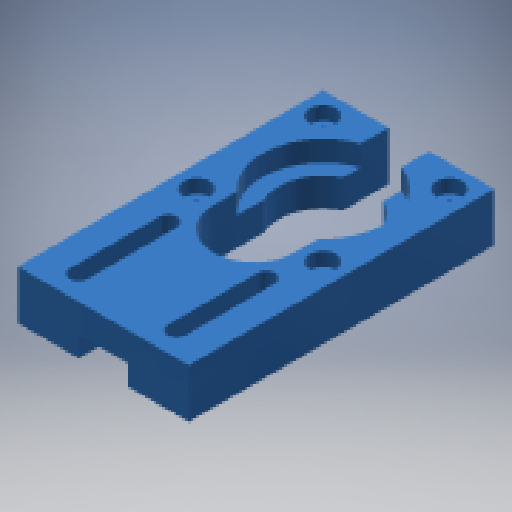
# Autodesk Inventor part: 24_0497_008
Saved by Autodesk Inventor 2024.3 (Build 283343000, 343)
## iProperties
Created: 2024-06-11
Part Number: 24_0497_008
Material: Allgemein
Document SubType Name: Modeling
Designer: Vogel
Density: 1 g/cm^3
Appearance: Cyan
Author: Vogel
Autodesk Inventor part; units mm, degrees
ref_plane "YZ Plane" through (0, 0, 0) normal (1, 0, 0) x (0, 1, 0)
ref_plane "XZ Plane" through (0, 0, 0) normal (0, 1, 0) x (-1, 0, 0)
ref_plane "XY Plane" through (0, 0, 0) normal (0, 0, 1) x (1, 0, 0)
sketch "Skizze1" plane through (0, 0, 0) normal (0, 0, 1) x (1, 0, 0)
  line L0 (-29.4, 0) -> (29.4, 0) projected
  line L1 (0, -69) -> (0, 36) projected
  line L2 (21, -54) -> (-21, -54)
  line L3 (-21, -54) -> (-21, 21)
  line L4 (-21, 21) -> (21, 21)
  line L5 (21, 21) -> (21, -54)
  line L6 (21, -54) -> (-21, 21) construction
  line L7 (-21, -54) -> (21, 21) construction
  circle A0 centre (0, 0) radius 11
  point P0 (0, -16.5)
  dimension "d0" = 42
  dimension "d1" = 75
  dimension "d3" = 22
  dimension "d4" = 21
  constraints: 12 end point, 3 midpoint, 2 parallel, 1 centre point, 1 coincident, 1 horizontal, 1 perpendicular
  measures "d0" distance of L3.end L4.end
  measures "d1" distance of L2.end L3.end
  measures "d3" diameter of A0
  measures "d4" distance between parallel lines of L0 L4
extrude "Extrusion1" add sketch "Skizze1" along normal blind 12 contours L3 L4 L1 A0 L0 | L0 A0 L1 L2 L3 | L1 L4 L5 L0 A0 | A0 L0 L5 L2 L1
sketch "Skizze2" plane through (0, 0, 12) normal (0, 0, 1) x (1, 0, 0)
  line L0 (21, -54) -> (21, 21) projected
  line L1 (21, 21) -> (-21, 21) projected
  line L2 (-21, 21) -> (-21, -54) projected
  line L3 (-21, -54) -> (21, -54) projected
  circle A0 centre (0, 0) radius 11 projected
  line L4 (15.5, -15.5) -> (-15.5, -15.5)
  line L5 (-15.5, -15.5) -> (-15.5, 15.5)
  line L6 (-15.5, 15.5) -> (15.5, 15.5)
  line L7 (15.5, 15.5) -> (15.5, -15.5)
  line L8 (15.5, -15.5) -> (-15.5, 15.5) construction
  line L9 (-15.5, -15.5) -> (15.5, 15.5) construction
  dimension "d7" = 31
  dimension "d8" = 31
  constraints: 12 end point, 4 coincident, 2 midpoint, 2 parallel, 1 horizontal, 1 perpendicular
  measures "d7" distance of L5.end L6.end
  measures "d8" distance of L4.end L5.end
hole "Bohrung1" at (-15.5, 15.5, 12) at (15.5, 15.5, 12) at (15.5, -15.5, 12) at (-15.5, -15.5, 12) direction (0, 0, -1) diameter 3.4 end through all counterbore diameter 6.5 counterbore depth 3.4
sketch "Skizze3" plane through (0, 0, 0) normal (0, 0, -1) x (-1, 0, 0)
  circle A0 centre (15.5, -15.5) radius 1.7 projected
  circle A1 centre (-15.5, -15.5) radius 1.7 projected
  circle A2 centre (-15.5, 15.5) radius 1.7 projected
  circle A3 centre (15.5, 15.5) radius 1.7 projected
  line L0 (-21, -54) -> (-21, 21) projected
  line L1 (21, -54) -> (-21, -54) projected
  line L2 (21, 21) -> (21, -54) projected
  line L3 (-21, 21) -> (21, 21) projected
  circle A4 centre (0, 0) radius 11 projected
  line L4 (29.4, 0) -> (-29.4, 0) projected
  line L5 (0, -69) -> (0, 36) projected
  line L6 (-12, -48) -> (-12, -26) construction
  line L7 (-8, -48) -> (-8, -26)
  line L8 (-16, -26) -> (-16, -48)
  arc A5 (-16, -48) -> (-8, -48) centre (-12, -48) ccw
  arc A6 (-8, -26) -> (-16, -26) centre (-12, -26) ccw
  line L9 (12, -48) -> (12, -26) construction
  line L10 (16, -48) -> (16, -26)
  line L11 (8, -26) -> (8, -48)
  arc A7 (8, -48) -> (16, -48) centre (12, -48) ccw
  arc A8 (16, -26) -> (8, -26) centre (12, -26) ccw
  point P0 (-12, -37)
  point P1 (12, -37)
  dimension "d16" = 24
  dimension "d17" = 8
  dimension "d18" = 8
  dimension "d19" = 6
  dimension "d20" = 22
  constraints: 16 end point, 8 point on circle, 8 tangent, 4 centre point, 3 parallel, 2 horizontal alignment, 2 midpoint, 1 vertical, 1 other
  measures "d16" distance between parallel lines of L6 L9
  measures "d17" distance between parallel lines of L8 L7
  measures "d18" distance between parallel lines of L11 L10
  measures "d19" distance from line of L1 L9.start
  measures "d20" distance of L8.start L8.end
extrude "Extrusion2" cut sketch "Skizze3" against normal blind 5 contours A5 L8 A6 L7 | A7 L11 A8 L10
sketch "Skizze4" plane through (0, 0, 0) normal (0, 0, -1) x (-1, 0, 0)
  arc A0 (-8, -26) -> (-16, -26) centre (-12, -26) ccw projected
  line L0 (-16, -48) -> (-16, -26) projected
  arc A1 (-16, -48) -> (-8, -48) centre (-12, -48) ccw projected
  line L1 (-8, -26) -> (-8, -48) projected
  arc A2 (16, -26) -> (8, -26) centre (12, -26) ccw projected
  line L2 (8, -48) -> (8, -26) projected
  arc A3 (8, -48) -> (16, -48) centre (12, -48) ccw projected
  line L3 (16, -26) -> (16, -48) projected
  line L4 (12, -48) -> (12, -26) construction
  line L5 (14.2, -48) -> (14.2, -26)
  line L6 (9.8, -26) -> (9.8, -48)
  arc A4 (9.8, -48) -> (14.2, -48) centre (12, -48) ccw
  arc A5 (14.2, -26) -> (9.8, -26) centre (12, -26) ccw
  line L7 (-12, -48) -> (-12, -26) construction
  line L8 (-9.8, -48) -> (-9.8, -26)
  line L9 (-14.2, -26) -> (-14.2, -48)
  arc A6 (-14.2, -48) -> (-9.8, -48) centre (-12, -48) ccw
  arc A7 (-9.8, -26) -> (-14.2, -26) centre (-12, -26) ccw
  point P0 (0, 0)
  point P1 (12, -37)
  point P2 (-12, -37)
  dimension "d23" = 4.4
  dimension "d24" = 4.4
  constraints: 16 end point, 8 point on circle, 8 tangent, 4 centre point, 4 parallel, 2 midpoint
  measures "d23" distance between parallel lines of L6 L5
  measures "d24" distance between parallel lines of L9 L8
extrude "Extrusion3" cut sketch "Skizze4" against normal through all contours A4 L6 A5 L5 | A6 L9 A7 L8
sketch "Skizze5" plane through (0, 0, 12) normal (0, 0, 1) x (1, 0, 0)
  line L0 (-9.8, -26) -> (-9.8, -48) projected
  arc A0 (-14.2, -48) -> (-9.8, -48) centre (-12, -48) ccw projected
  line L1 (-14.2, -48) -> (-14.2, -26) projected
  arc A1 (-9.8, -26) -> (-14.2, -26) centre (-12, -26) ccw projected
  line L2 (14.2, -26) -> (14.2, -48) projected
  arc A2 (9.8, -48) -> (14.2, -48) centre (12, -48) ccw projected
  line L3 (9.8, -48) -> (9.8, -26) projected
  arc A3 (14.2, -26) -> (9.8, -26) centre (12, -26) ccw projected
  circle A4 centre (-15.5, -15.5) radius 3.25 projected
  circle A5 centre (15.5, -15.5) radius 3.25 projected
  circle A6 centre (15.5, 15.5) radius 3.25 projected
  circle A7 centre (-15.5, 15.5) radius 3.25 projected
  line L4 (21, -54) -> (21, 21) projected
  line L5 (21, 21) -> (-21, 21) projected
  line L6 (-21, 21) -> (-21, -54) projected
  line L7 (-21, -54) -> (21, -54) projected
  circle A8 centre (0, 0) radius 11 projected
  circle A9 centre (0, 0) radius 15
  dimension "d27" = 30
  constraints: 1 centre point, 1 coincident
  measures "d27" diameter of A9
extrude "Extrusion4" cut sketch "Skizze5" against normal blind 5 contours A9
sketch "Skizze6" plane through (0, 0, 12) normal (0, 0, 1) x (1, 0, 0)
  circle A0 centre (0, 0) radius 15 projected
  line L0 (-9.8, -26) -> (-9.8, -48) projected
  arc A1 (-14.2, -48) -> (-9.8, -48) centre (-12, -48) ccw projected
  line L1 (-14.2, -48) -> (-14.2, -26) projected
  arc A2 (-9.8, -26) -> (-14.2, -26) centre (-12, -26) ccw projected
  line L2 (14.2, -26) -> (14.2, -48) projected
  arc A3 (9.8, -48) -> (14.2, -48) centre (12, -48) ccw projected
  line L3 (9.8, -48) -> (9.8, -26) projected
  arc A4 (14.2, -26) -> (9.8, -26) centre (12, -26) ccw projected
  circle A5 centre (-15.5, -15.5) radius 3.25 projected
  circle A6 centre (15.5, -15.5) radius 3.25 projected
  circle A7 centre (15.5, 15.5) radius 3.25 projected
  circle A8 centre (-15.5, 15.5) radius 3.25 projected
  line L4 (21, -54) -> (21, 21) projected
  line L5 (21, 21) -> (-21, 21) projected
  line L6 (-21, 21) -> (-21, -54) projected
  line L7 (-21, -54) -> (21, -54) projected
  line L8 (-29.4, 0) -> (29.4, 0) projected
  line L9 (0, -69) -> (0, 36) projected
  line L10 (-5, 8) -> (5, 8)
  line L11 (5, 8) -> (5, 26)
  line L12 (5, 26) -> (-5, 26)
  line L13 (-5, 26) -> (-5, 8)
  line L14 (-5, 8) -> (5, 26) construction
  line L15 (5, 8) -> (-5, 26) construction
  point P0 (0, 17)
  dimension "d30" = 18
  dimension "d31" = 10
  dimension "d32" = 8
  constraints: 12 end point, 2 midpoint, 2 parallel, 1 horizontal, 1 perpendicular, 1 point on line
  measures "d30" distance of L12.end L10.start
  measures "d31" distance of L11.end L12.end
  measures "d32" distance between parallel lines of L8 L10
extrude "Extrusion5" cut sketch "Skizze6" against normal through all contours L11 L10 L9 A0 | A0 L9 L5 L11 | L9 L10 L13 A0 | A0 L13 L5 L9 | L5 L9 L12 L11 | L5 L13 L12 L9
sketch "Skizze7" plane through (0, 0, 12) normal (0, 0, 1) x (1, 0, 0)
  line L0 (5, 14.1421) -> (5, 9.798) projected
  arc A0 (-5, 9.798) -> (5, 9.798) centre (0, 0) ccw projected
  line L1 (-5, 9.798) -> (-5, 14.1421) projected
  arc A1 (-5, 14.1421) -> (5, 14.1421) centre (0, 0) ccw projected
  line L2 (-29.4, 0) -> (29.4, 0) projected
  line L3 (0, -69) -> (0, 36) projected
  line L4 (0, 0) -> (0, -17) construction
  line L5 (-10, 0) -> (-10, -17)
  line L6 (10, -17) -> (10, 0)
  arc A2 (10, 0) -> (-10, 0) centre (0, 0) ccw
  arc A3 (-10, -17) -> (10, -17) centre (0, -17) ccw
  point P0 (0, -8.5)
  dimension "d35" = 20
  dimension "d36" = 17
  constraints: 8 end point, 4 point on circle, 4 tangent, 2 centre point, 1 midpoint, 1 parallel, 1 point on line
  measures "d35" distance between parallel lines of L5 L6
  measures "d36" distance of L5.start L5.end
extrude "Extrusion6" cut sketch "Skizze7" against normal through all contours L6 A3 L3 A1 | A1 L3 A0 L6 | A0 L3 L2 L6 | L2 L3 A2 | L3 A3 L5 A1 | A1 L5 A0 L3 | A0 L5 L2 L3 | L2 A2 L3
sketch "Skizze8" plane through (0, 0, 0) normal (0, 0, -1) x (-1, 0, 0)
  line L0 (-5, 9.798) -> (-5, 21) projected
  line L1 (-21, 21) -> (-5, 21) projected
  line L2 (-21, -54) -> (-21, 21) projected
  line L3 (21, -54) -> (-21, -54) projected
  line L4 (21, 21) -> (21, -54) projected
  line L5 (5, 21) -> (21, 21) projected
  line L6 (5, 21) -> (5, 9.798) projected
  arc A0 (-5, 9.798) -> (-10, -4.5826) centre (0, 0) ccw projected
  circle A1 centre (15.5, 15.5) radius 1.7 projected
  circle A2 centre (-15.5, 15.5) radius 1.7 projected
  circle A3 centre (-15.5, -15.5) radius 1.7 projected
  circle A4 centre (15.5, -15.5) radius 1.7 projected
  line L7 (-16, -48) -> (-16, -26) projected
  arc A5 (-8, -26) -> (-16, -26) centre (-12, -26) ccw projected
  line L8 (-8, -26) -> (-8, -48) projected
  arc A6 (-16, -48) -> (-8, -48) centre (-12, -48) ccw projected
  line L9 (8, -48) -> (8, -26) projected
  arc A7 (16, -26) -> (8, -26) centre (12, -26) ccw projected
  line L10 (16, -26) -> (16, -48) projected
  arc A8 (8, -48) -> (16, -48) centre (12, -48) ccw projected
  line L11 (29.4, 0) -> (-29.4, 0) projected
  line L12 (0, -69) -> (0, 36) projected
  line L13 (10, -4.5826) -> (10, -17) projected
  arc A9 (-10, -17) -> (10, -17) centre (0, -17) ccw projected
  line L14 (-10, -17) -> (-10, -4.5826) projected
  arc A10 (10, -4.5826) -> (5, 9.798) centre (0, 0) ccw projected
  line L15 (0, 0) -> (0, -60) construction
  line L16 (-6, 0) -> (-6, -60)
  line L17 (6, -60) -> (6, 0)
  arc A11 (6, 0) -> (-6, 0) centre (0, 0) ccw
  arc A12 (-6, -60) -> (6, -60) centre (0, -60) ccw
  point P0 (0, -30)
  point P1 (11, 0)
  point P2 (21, 0)
  point P3 (-21, 0)
  point P4 (-11, 0)
  point P5 (-6, -25)
  point P6 (6, -25)
  point P7 (0, -66)
  point P8 (0, -54)
  point P9 (-6, -54)
  point P10 (0, 6)
  point P11 (0, -27)
  point P12 (6, -54)
  dimension "d39" = 12
  dimension "d40" = 60
  constraints: 8 end point, 4 point on circle, 4 tangent, 2 centre point, 1 midpoint, 1 parallel, 1 point on line, 1 other
  measures "d39" distance between parallel lines of L16 L17
  measures "d40" distance of L17.start L17.end
extrude "Extrusion7" cut sketch "Skizze8" against normal blind 5 contours A11 L12 L11 | L11 L12 A9 L16 | L12 A11 L11 | L11 L17 A9 L12 | A9 L12 L3 L16 | A9 L17 L3 L12 | L3 L12 A12 L16 | L3 L17 A12 L12
equation "\"d18\" = d17"
equation "\"d24\" = d23"
